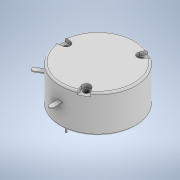
# Autodesk Inventor part: S200 EChem Sensor
Saved by Autodesk Inventor 2021 (Build 250183000, 183)
## iProperties
Created: 2020-07-06
Part Number: S200 EChem Sensor
Material: Generic
Document SubType Name: Modeling
Designer: jgray
Density: 1 g/cm^3
Appearance: Default
Author: jgray
Autodesk Inventor part; units mm, degrees
ref_plane "YZ Plane" through (0, 0, 0) normal (1, 0, 0) x (0, 1, 0)
ref_plane "XZ Plane" through (0, 0, 0) normal (0, 1, 0) x (-1, 0, 0)
sketch "Sketch1" plane through (0, 0, 0) normal (0, 1, 0) x (-1, 0, 0)
  circle A0 centre (0, 0) radius 20.5
  dimension "d0" = 41
  constraints: 1 centre point, 1 coincident
  measures "d0" diameter of A0
extrude "Extrusion1" add sketch "Sketch1" along normal blind 20.4
sketch "Sketch2" plane through (0, 20.4, 0) normal (0, 1, 0) x (1, 0, 0)
  line L0 (-25.2236, 0) -> (25.6343, 0)
  circle A0 centre (0, 0) radius 17.2 construction
  point P0 (-17.2, 0)
  point P1 (8.6, -14.8956)
  point P2 (8.6, 14.8956)
  dimension "d3" = 34.4
  dimension "d6" = 360
  constraints: 2 end point, 2 point on line, 1 coincident, 1 horizontal, 1 horizontal alignment, 6 other
hole "Hole1" at (-17.2, 20.4, 0) at (8.6, 20.4, 14.8956) at (8.6, 20.4, -14.8956) direction (0, -1, 0) diameter 3 end through all counterbore diameter 4.4 counterbore depth 2
sketch "Sketch3" plane through (0, 20.4, 0) normal (0, 1, 0) x (1, 0, 0)
  circle A0 centre (8.6, -14.8956) radius 2.2 projected
  circle A1 centre (-17.2, 0) radius 2.2 projected
  circle A2 centre (8.6, 14.8956) radius 2.2 projected
  circle A3 centre (0, 0) radius 20.5 projected
  line L0 (6.5697, -15.7429) -> (7.895, -18.9187)
  circle A4 centre (0, 0) radius 20.5 projected
  line L1 (10.3489, -13.561) -> (12.4366, -16.2966)
  line L2 (10.3489, 13.561) -> (12.4366, 16.2966)
  line L3 (6.5697, 15.7429) -> (7.895, 18.9187)
  line L4 (-16.9186, 2.1819) -> (-20.3316, 2.6221)
  line L5 (-16.9186, -2.1819) -> (-20.3316, -2.6221)
  circle A5 centre (-17.2, 0) radius 2.2 projected
  circle A6 centre (8.6, 14.8956) radius 2.2 projected
  circle A7 centre (8.6, -14.8956) radius 2.2 projected
  constraints: 12 end point, 12 point on circle, 6 tangent
extrude "Extrusion2" cut sketch "Sketch3" against normal blind 2 contours A0 L1 A3 L0 | A3 L4 A1 L5 | L2 A2 L3 A3
ref_plane "Work Plane1" through (0, 12.4, 0) normal (0, 1, 0) x (1, 0, 0)
sketch "Sketch4" plane through (0, 12.4, 0) normal (0, 1, 0) x (1, 0, 0)
  circle A0 centre (8.6, -14.8956) radius 1.5 projected
  circle A1 centre (-17.2, 0) radius 1.5 projected
  circle A2 centre (8.6, 14.8956) radius 1.5 projected
  circle A3 centre (0, 0) radius 20.5 projected
  line L0 (0, 0) -> (-21.2105, -12.2459) construction
  line L1 (0, 0) -> (-21.8671, 12.625) construction
  line L2 (-23.6336, 0) -> (24.9961, 0) construction
  line L3 (0, 0) -> (0, -27.2781) construction
  line L4 (-12.9995, 7.5053) -> (-21.8671, 12.625) construction
  line L5 (-12.3745, 8.5878) -> (-21.2421, 13.7075)
  line L6 (-22.4921, 11.5425) -> (-13.6245, 6.4228)
  arc A4 (-13.6245, 6.4228) -> (-12.3745, 8.5878) centre (-12.9995, 7.5053) ccw
  arc A5 (-21.2421, 13.7075) -> (-22.4921, 11.5425) centre (-21.8671, 12.625) ccw
  line L7 (-21.8671, -12.625) -> (-13.5975, -7.8505) construction
  line L8 (-21.2421, -13.7075) -> (-12.9725, -8.9331)
  line L9 (-14.2225, -6.768) -> (-22.4921, -11.5425)
  arc A6 (-22.4921, -11.5425) -> (-21.2421, -13.7075) centre (-21.8671, -12.625) ccw
  arc A7 (-12.9725, -8.9331) -> (-14.2225, -6.768) centre (-13.5975, -7.8505) ccw
  line L10 (0, -25.25) -> (0, -15.6538) construction
  line L11 (1.25, -25.25) -> (1.25, -15.6538)
  line L12 (-1.25, -15.6538) -> (-1.25, -25.25)
  arc A8 (-1.25, -25.25) -> (1.25, -25.25) centre (0, -25.25) ccw
  arc A9 (1.25, -15.6538) -> (-1.25, -15.6538) centre (0, -15.6538) ccw
  point P0 (-17.4333, 10.0651)
  point P1 (-17.7323, -10.2378)
  point P2 (0, -20.4519)
  point P3 (-18.3455, 9.1484)
  point P4 (-17.0955, 11.3135)
  dimension "d18" = 30
  dimension "d19" = 30
  dimension "d20" = 60
  dimension "d21" = 2.5
  dimension "d22" = 6
  dimension "d23" = 2.5
  dimension "d24" = 2.5
  dimension "d25" = 6
  dimension "d26" = 6
  constraints: 32 end point, 12 point on circle, 12 tangent, 6 centre point, 5 point on line, 3 midpoint, 3 parallel, 1 collinear, 1 horizontal
  measures "d18" angle of L2 L0
  measures "d19" angle of L2 L1
  measures "d20" angle of L3 L0
  measures "d21" diameter of A5
  measures "d23" diameter of A7
  measures "d24" diameter of A9
extrude "Extrusion3" add sketch "Sketch4" against normal blind 0.5 contours A3 L6 A5 L5 | L11 A8 L12 A3 | A3 L12 A9 L11 | L9 A7 L8 A3 | A3 L8 A6 L9
sketch "Sketch5" plane through (0, 0, 0) normal (0, -1, 0) x (1, 0, 0)
  arc A0 (-17.0955, 11.3135) -> (-18.3455, 9.1484) centre (0, 0) ccw projected
  line L0 (-17.0955, 11.3135) -> (-21.2421, 13.7075) projected
  arc A1 (-21.2421, 13.7075) -> (-22.4921, 11.5425) centre (-21.8671, 12.625) ccw projected
  line L1 (-22.4921, 11.5425) -> (-18.3455, 9.1484) projected
  line L2 (-18.3455, -9.1484) -> (-22.4921, -11.5425) projected
  arc A2 (-22.4921, -11.5425) -> (-21.2421, -13.7075) centre (-21.8671, -12.625) ccw projected
  line L3 (-21.2421, -13.7075) -> (-17.0955, -11.3135) projected
  arc A3 (-18.3455, -9.1484) -> (-17.0955, -11.3135) centre (0, 0) ccw projected
  arc A4 (1.25, 20.4619) -> (-1.25, 20.4619) centre (0, 0) ccw projected
  line L4 (1.25, 20.4619) -> (1.25, 25.25) projected
  arc A5 (1.25, 25.25) -> (-1.25, 25.25) centre (0, 25.25) ccw projected
  line L5 (-1.25, 25.25) -> (-1.25, 20.4619) projected
  circle A6 centre (8.6, 14.8956) radius 1.5 projected
  circle A7 centre (-17.2, 0) radius 1.5 projected
  circle A8 centre (8.6, -14.8956) radius 1.5 projected
  circle A9 centre (0, 0) radius 20.5 projected
  line L6 (0, 34.5014) -> (0, -27.9837) construction
  line L7 (0, 0) -> (-32.677, 18.8661) construction
  line L8 (0, 0) -> (-32.677, -18.8661) construction
  circle A10 centre (0, 0) radius 17.2 construction
  circle A11 centre (0, 17.2) radius 1.5
  circle A12 centre (-14.8956, 8.6) radius 1.5
  circle A13 centre (-14.8956, -8.6) radius 1.5
  dimension "d29" = 34.4
  dimension "d30" = 3
  dimension "d31" = 3
  dimension "d32" = 3
  constraints: 9 point on line, 6 end point, 4 centre point, 3 point on circle, 1 coincident, 1 parallel, 1 vertical
  measures "d29" diameter of A10
  measures "d30" diameter of A11
  measures "d31" diameter of A12
  measures "d32" diameter of A13
extrude "Extrusion4" cut sketch "Sketch5" against normal blind 0.2 contours A11 | A12 | A13
sketch "Sketch7" plane through (-14.8956, 0.2, 8.6) normal (0, -1, 0) x (1, 0, 0)
  circle A0 centre (14.8956, 8.6) radius 1.5 projected
  circle A1 centre (0, 0) radius 1.5 projected
  circle A2 centre (0, -17.2) radius 1.5 projected
  circle A3 centre (23.4956, 6.2956) radius 1.5 projected
  circle A4 centre (-2.3044, -8.6) radius 1.5 projected
  circle A5 centre (23.4956, -23.4956) radius 1.5 projected
  circle A6 centre (14.8956, -8.6) radius 20.5 projected
  circle A7 centre (0, 0) radius 0.5
  circle A8 centre (14.8956, 8.6) radius 0.5
  circle A9 centre (0, -17.2) radius 0.5
  dimension "d36" = 1
  dimension "d37" = 1
  dimension "d38" = 1
  constraints: 3 centre point, 3 coincident
  measures "d36" diameter of A7
  measures "d37" diameter of A8
  measures "d38" diameter of A9
extrude "Extrusion5" add sketch "Sketch7" along normal blind 4.5 contours A7 | A8 | A9
fillet "Fillet1" radius 0.5 3 edges at (-15.3956, -4.3, -8.6) (-15.3956, -4.3, 8.6) (-0.5, -4.3, 17.2)
fillet "Fillet2" radius 1 4 edges at (-10.25, 20.4, 17.7535) (-10.25, 20.4, -17.7535) (20.5, 20.4, 0) (20.5, 0, 0)
body "Solid1"
